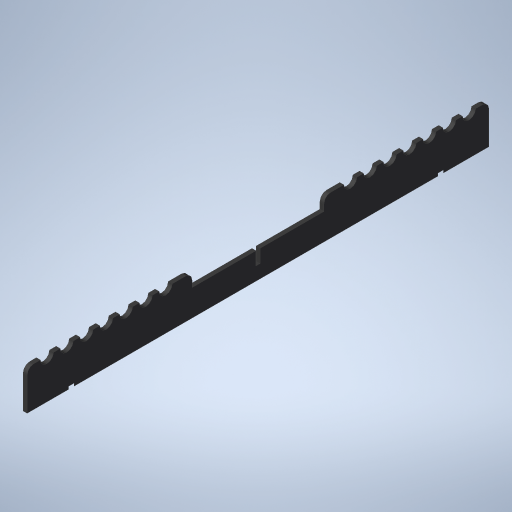
# Autodesk Inventor part: StoveTop2
Saved by Autodesk Inventor 2024.3 (Build 283343000, 343)
## iProperties
Created: 2025-06-28
Part Number: StoveTop2
Material: Generic
Document SubType Name: Modeling
Designer: ajclo
Density: 1 g/cm^3
Appearance: Default
Author: ajclo
Autodesk Inventor part; units mm, degrees
ref_plane "YZ Plane" through (0, 0, 0) normal (1, 0, 0) x (0, 1, 0)
ref_plane "XZ Plane" through (0, 0, 0) normal (0, 1, 0) x (-1, 0, 0)
ref_plane "XY Plane" through (0, 0, 0) normal (0, 0, 1) x (1, 0, 0)
sketch "Sketch1" plane through (0, 0, 0) normal (1, 0, 0) x (0, 1, 0)
  line L0 (0, 175) -> (30, 175)
  line L1 (30, 175) -> (30, -175)
  line L2 (30, -175) -> (0, -175)
  line L3 (0, -175) -> (0, 175)
  line L4 (40, 50) -> (20, 50)
  line L5 (20, 50) -> (20, -50)
  line L6 (20, -50) -> (40, -50)
  line L7 (40, -3.1) -> (40, 50)
  line L8 (40, 50) -> (20, -50) construction
  line L9 (20, 50) -> (40, -50) construction
  line L10 (30, 1.55) -> (10, 1.55)
  line L11 (10, 1.55) -> (10, -1.55)
  line L12 (30, -1.55) -> (30, 1.55)
  line L13 (30, 1.55) -> (10, -1.55) construction
  line L14 (10, 1.55) -> (30, -1.55) construction
  line L15 (10, -1.55) -> (20, -1.55)
  line L16 (29.69, -1.55) -> (30, -1.55)
  point P0 (0, 0)
  point P1 (0, 0)
  point P2 (30, 0)
  point P3 (20, 0)
  point P4 (30, -50)
  point P5 (20, 1.55)
  point P6 (30, 50)
  dimension "d0" = 30
  dimension "d1" = 350
  dimension "d2" = 0
  dimension "d3" = 100
  dimension "d4" = 20
  dimension "d5" = 20
  dimension "d6" = 3.1
  constraints: 34 end point, 7 midpoint, 7 parallel, 3 horizontal, 3 perpendicular, 3 point on line
  measures "d0" distance of L0.start L0.end
  measures "d1" distance of L0.end L1.end
  measures "d2" distance of point (0, 0) point (0, 0)
  measures "d3" distance of L4.end L5.end
  measures "d4" distance of L5.end L6.end
  measures "d5" distance of L11.end L12.start
  measures "d6" distance of L10.end L11.end
extrude "Extrusion1" add sketch "Sketch1" along normal blind 3 contours L0 L1 L4 L5 L10 L11 L15 L6 L2 L3
sketch "Sketch2" plane through (3, 0, 0) normal (1, 0, 0) x (0, 0, -1)
  line L0 (-50, 30) -> (-175, 30) projected
  circle A0 centre (-160, 30) radius 5
  circle A1 centre (-145, 30) radius 5
  circle A2 centre (-130, 30) radius 5
  circle A3 centre (-115, 30) radius 5
  circle A4 centre (-100, 30) radius 5
  circle A5 centre (-85, 30) radius 5
  circle A6 centre (-70, 30) radius 5
  line L1 (-175, 30) -> (-175, 0) projected
  line L2 (-50, 30) -> (-175, 30) projected
  point P0 (0, 0)
  point P1 (-75, 30)
  point P2 (-65, 30)
  point P3 (-90, 30)
  point P4 (-80, 30)
  point P5 (-105, 30)
  point P6 (-95, 30)
  point P7 (-120, 30)
  point P8 (-110, 30)
  point P9 (-135, 30)
  point P10 (-125, 30)
  point P11 (-150, 30)
  point P12 (-140, 30)
  point P13 (-165, 30)
  point P14 (-155, 30)
  dimension "d9" = 10
  dimension "d10" = 10
  dimension "d11" = 10
  dimension "d12" = 10
  dimension "d13" = 10
  dimension "d14" = 10
  dimension "d15" = 10
  dimension "d16" = 15
  dimension "d17" = 15
  dimension "d18" = 15
  dimension "d19" = 15
  dimension "d20" = 15
  dimension "d21" = 15
  dimension "d22" = 15
  constraints: 7 centre point, 1 point on line, 7 other
  measures "d9" diameter of A0
  measures "d10" diameter of A1
  measures "d11" diameter of A2
  measures "d12" diameter of A3
  measures "d13" diameter of A4
  measures "d14" diameter of A5
  measures "d15" diameter of A6
  measures "d16" distance of A1.centre A0.centre
  measures "d17" distance from line of L1 A0.centre
  measures "d18" distance of A1.centre A2.centre
  measures "d19" distance of A3.centre A2.centre
  measures "d20" distance of A4.centre A3.centre
  measures "d21" distance of A5.centre A4.centre
  measures "d22" distance of A5.centre A6.centre
extrude "Extrusion2" cut sketch "Sketch2" against normal blind 3 contours A6 L0 | A5 L0 | A4 L0 | A3 L0 | A2 L0 | A1 L0 | A0 L0 picked at (-68.8623, 27.8538) picked at (-83.8623, 27.8538) picked at (-98.8623, 27.8538) picked at (-113.8623, 27.8538) picked at (-131.2475, 28.8948) picked at (-146.4384, 28.1203) picked at (-161.4384, 28.1203)
fillet "Fillet1" radius 5 2 edges at (1.5, 30, 175) (1.5, 30, 50)
mirror "Mirror1" about plane through (0, 0, 0) normal (0, 0, 1) of "Fillet1", "Extrusion2"
sketch "Sketch3" plane through (0, 0, -175) normal (0, -1, 0) x (1, 0, 0)
  line L0 (0, 350) -> (0, 0) projected
  line L1 (0, 0) -> (3, 0) projected
  line L2 (3, 350) -> (3, 0) projected
  line L3 (0, 350) -> (3, 350) projected
  line L4 (0, 315.6285) -> (3, 318.6285)
  line L5 (0, 311.3858) -> (3, 314.3858)
  line L6 (0, 35.6142) -> (3, 38.6142)
  line L7 (0, 31.3715) -> (3, 34.3715)
  line L8 (0, 175) -> (3, 175)
  point P0 (1.5, 175)
  dimension "d26" = 3
  dimension "d27" = 45
  dimension "d28" = 3
  dimension "d29" = 195
  dimension "d33" = 97.5
  constraints: 10 end point, 8 point on line, 3 midpoint, 3 parallel
  measures "d26" distance between parallel lines of L7 L6
  measures "d27" angle of L0 L6
  measures "d28" distance between parallel lines of L5 L4
  measures "d29" distance between parallel lines of L5 L6
  measures "d33" distance from line of point (1.5, 175) L6
extrude "Extrusion3" cut sketch "Sketch3" against normal blind 2 contours L4 L2 L5 L0 | L6 L2 L7 L0
equation "\"d10\" = d9"
equation "\"d11\" = d10"
equation "\"d12\" = d9"
equation "\"d13\" = d9"
equation "\"d14\" = d9"
equation "\"d15\" = d9"
equation "\"d20\" = d19"
equation "\"d21\" = d20"
equation "\"d22\" = d21"
body "Solid1"
